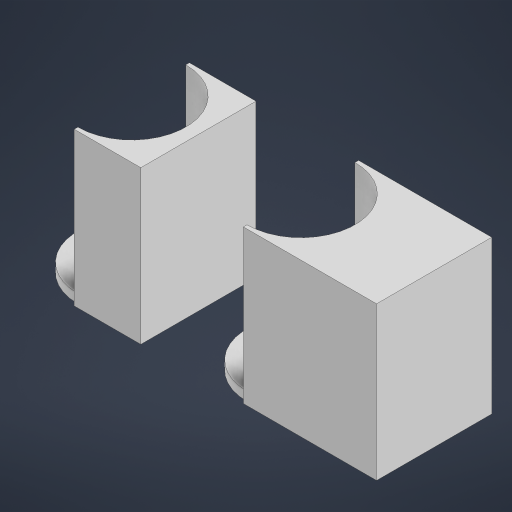
# Autodesk Inventor part: motor-holders
Saved by Autodesk Inventor 2023 (Build 270158030, 158C)
## iProperties
Created: 2022-05-28
Part Number: motor-holders
Material: Generic
Document SubType Name: Modeling
Designer: jayso
Density: 1 g/cm^3
Appearance: Default
Author: jayso
Autodesk Inventor part; units mm, degrees
ref_plane "YZ Plane" through (0, 0, 0) normal (1, 0, 0) x (0, 1, 0)
ref_plane "XZ Plane" through (0, 0, 0) normal (0, 1, 0) x (-1, 0, 0)
ref_plane "XY Plane" through (0, 0, 0) normal (0, 0, 1) x (1, 0, 0)
sketch "Sketch2" plane through (0, 0, 0) normal (0, 1, 0) x (-1, 0, 0)
  line L0 (49.5, 16) -> (-49.5, 16)
  line L1 (-49.5, 16) -> (-49.5, -16)
  line L2 (-49.5, -16) -> (49.5, -16)
  line L3 (49.5, -16) -> (49.5, 16)
  circle A0 centre (-12.5, 0) radius 15
  circle A1 centre (34.5, 0) radius 15
  line L4 (16, 16) -> (-12.5, 16)
  line L5 (-12.5, 16) -> (-12.5, -16)
  line L6 (-12.5, -16) -> (16, -16)
  line L7 (16, -16) -> (16, 16)
  line L8 (49.5, 16) -> (34.5, 16)
  line L9 (34.5, 16) -> (34.5, -16)
  line L10 (34.5, -16) -> (49.5, -16)
  line L11 (49.5, -16) -> (49.5, 16)
  point P0 (0, 0)
  point P1 (49.5, 0)
  point P2 (34.5, 15)
  point P3 (34.5, -15)
  point P4 (-12.5, -15)
  point P5 (-12.5, 15)
  dimension "d0" = 99
  dimension "d1" = 32
  dimension "d2" = 16
  dimension "d3" = 49.5
  dimension "d6" = 30
  dimension "d7" = 37
  dimension "d8" = 30
  dimension "d9" = 47
  dimension "d10" = 28.5
  dimension "d11" = 0
  constraints: 24 end point, 6 parallel, 3 horizontal, 3 perpendicular, 3 point on line, 2 centre point, 1 midpoint
  measures "d0" distance of L1.end L2.end
  measures "d1" distance of L0.end L1.end
  measures "d2" distance from line of point (0, 0) L2
  measures "d3" distance of point (0, 0) point (49.5, 0)
  measures "d6" diameter of A0
  measures "d7" distance from line of L1 A0.centre
  measures "d8" diameter of A1
  measures "d9" distance of A0.centre A1.centre
  measures "d10" distance of L5.end L6.end
  measures "d11" distance from line of A0.centre L5
extrude "Extrusion2" add sketch "Sketch2" along normal blind 42.5 contours L9 A1 L2 L7 L0 | L5 A0 L2 L1 L0
extrude "Extrusion3" add sketch "Sketch2" along normal blind 2.5 separate body contours A1 L9 | L9 A1 | L5 A0 | A0 L5
combine bodies "Combine1" operation type add bodies to combine 1 2
body "Solid3"
